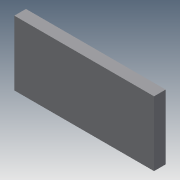
# Autodesk Inventor part: servodrzak3
Saved by Autodesk Inventor 2013 (Build 170138000, 138)
## iProperties
Created: 2013-01-30
Part Number: servodrzak3
Material: Generic
Document SubType Name: Modeling
Designer: idle-rug
Density: 1 g/cm^3
Author: idle-rug
Autodesk Inventor part; units mm, degrees
ref_plane "YZ Plane" through (0, 0, 0) normal (1, 0, 0) x (0, 1, 0)
ref_plane "XZ Plane" through (0, 0, 0) normal (0, 1, 0) x (-1, 0, 0)
ref_plane "XY Plane" through (0, 0, 0) normal (0, 0, 1) x (1, 0, 0)
sketch "Sketch1" plane through (0, 0, 0) normal (0, 1, 0) x (-1, 0, 0)
  line L0 (30, 13.9) -> (-30, 13.9)
  line L1 (-30, 13.9) -> (-30, -13.9)
  line L2 (-30, -13.9) -> (30, -13.9)
  line L3 (30, -13.9) -> (30, 13.9)
  line L4 (30, 13.9) -> (-30, -13.9) construction
  line L5 (-30, 13.9) -> (30, -13.9) construction
  point P0 (0, 0)
  dimension "d0" = 60
  dimension "d1" = 27.8
  constraints: 12 end point, 2 midpoint, 2 parallel, 1 horizontal, 1 perpendicular
  measures "d0" distance of L2.end L1.end
  measures "d1" distance of L1.end L0.end
extrude "Extrusion1" add sketch "Sketch1" along normal blind 5
body "Solid1"
